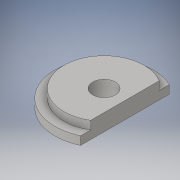
# Autodesk Inventor part: Spring Clamp Small
Saved by Autodesk Inventor 2016 (Build 200138000, 138)
## iProperties
Created: 2015-06-15
Part Number: Spring Clamp Small
Material: Generic
Document SubType Name: Modeling
Designer: Dennis
Density: 1 g/cm^3
Appearance: Default
Author: Dennis
Autodesk Inventor part; units mm, degrees
ref_plane "YZ Plane" through (0, 0, 0) normal (1, 0, 0) x (0, 1, 0)
ref_plane "XZ Plane" through (0, 0, 0) normal (0, 1, 0) x (-1, 0, 0)
ref_plane "XY Plane" through (0, 0, 0) normal (0, 0, 1) x (1, 0, 0)
sketch "Sketch1" plane through (0, 0, 0) normal (0, 1, 0) x (-1, 0, 0)
  circle A0 centre (0, 0) radius 11.9126
  dimension "d0" = 23.8252
  constraints: 1 centre point, 1 coincident
  measures "d0" diameter of A0
extrude "Extrusion1" add sketch "Sketch1" along normal blind 2.032
sketch "Sketch2" plane through (0, 2.032, 0) normal (0, 1, 0) x (1, 0, 0)
  circle A0 centre (0, 0) radius 9.7536
  dimension "d3" = 19.5072
  constraints: 1 centre point, 1 coincident
  measures "d3" diameter of A0
extrude "Extrusion2" add sketch "Sketch2" along normal blind 2.032
sketch "Sketch3" plane through (0, 4.064, 0) normal (0, 1, 0) x (1, 0, 0)
  circle A0 centre (0, 0) radius 2.75
  dimension "d6" = 5.5
  constraints: 1 centre point, 1 coincident
  measures "d6" diameter of A0
extrude "Extrusion3" cut sketch "Sketch3" against normal blind 4.064
sketch "Sketch4" plane through (0, 4.064, 0) normal (0, 1, 0) x (1, 0, 0)
  line L0 (17.8511, 14.0442) -> (5.08, 14.0442)
  line L1 (5.08, 14.0442) -> (5.08, -15.9032)
  line L2 (5.08, -15.9032) -> (17.8511, -15.9032)
  line L3 (17.8511, -15.9032) -> (17.8511, 14.0442)
  point P0 (0, 0)
  dimension "d9" = 5.08
  constraints: 8 end point, 2 parallel, 1 horizontal, 1 perpendicular
  measures "d9" distance from line of point (0, 0) L1
extrude "Extrusion4" cut sketch "Sketch4" against normal blind 4.064
body "Solid1"
